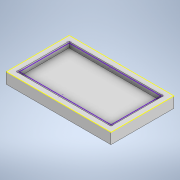
# Autodesk Inventor part: pan
Saved by Autodesk Inventor 2021 (Build 250183000, 183)
## iProperties
Created: 2021-07-07
Part Number: pan
Material: Generic
Document SubType Name: Modeling
Designer: Priyanka Hungund
Density: 1 g/cm^3
Appearance: Default
Author: Priyanka Hungund
Autodesk Inventor part; units mm, degrees
ref_plane "YZ Plane" through (0, 0, 0) normal (1, 0, 0) x (0, 1, 0)
ref_plane "XZ Plane" through (0, 0, 0) normal (0, 1, 0) x (-1, 0, 0)
ref_plane "XY Plane" through (0, 0, 0) normal (0, 0, 1) x (1, 0, 0)
sketch "Sketch1" plane through (0, 0, 0) normal (0, 0, 1) x (1, 0, 0)
  line L0 (-9.8509, 0) -> (10.5499, 0)
  line L1 (10.5499, 0) -> (10.5499, -2.1187)
  line L2 (10.5499, -2.1187) -> (-9.8509, -2.1187)
  line L3 (-9.8509, -2.1187) -> (-9.8509, 0)
  point P0 (0, 0)
  constraints: 8 end point, 2 parallel, 1 horizontal, 1 perpendicular
extrude "Extrusion1" add sketch "Sketch1" along normal blind 12.25
sketch "Sketch2" plane through (-9.8509, 0, 0) normal (0, 1, 0) x (1, 0, 0)
  line L0 (20.4008, 0) -> (0, 0) projected
  line L1 (0, 0) -> (0, -12.25) projected
  line L2 (20.4008, -12.25) -> (0, -12.25) projected
  line L3 (20.4008, 0) -> (20.4008, -12.25) projected
  line L4 (1.2669, -10.9831) -> (1.2669, -1.2669)
  line L5 (1.2669, -1.2669) -> (19.1339, -1.2669)
  line L6 (19.1339, -1.2669) -> (19.1339, -10.9831)
  line L7 (19.1339, -10.9831) -> (1.2669, -10.9831)
  point P0 (9.8509, 0)
  point P1 (9.3922, -1.2669)
  point P2 (9.3922, -10.9831)
  constraints: 8 end point, 4 coincident, 2 point on line, 3 other
shell "Shell1" thickness 1 removed faces 1 at (3.7496, 0, 4.0833)
body "Solid1"
